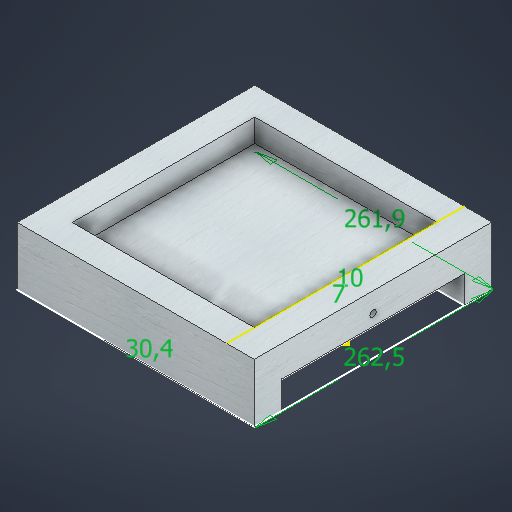
# Autodesk Inventor part: FundoColmeia
Saved by Autodesk Inventor 2027 (Build 310192000, 192)
## iProperties
Created: 2026-10-01
Part Number: FundoColmeia
Material: Genérico
Document SubType Name: Modeling
Designer: EspacoMaker
Density: 1 g/cm^3
Appearance: Padrão
Author: EspacoMaker
Autodesk Inventor part; units mm, degrees
ref_plane "YZ Plane" through (0, 0, 0) normal (1, 0, 0) x (0, 1, 0)
ref_plane "XZ Plane" through (0, 0, 0) normal (0, 1, 0) x (-1, 0, 0)
ref_plane "XY Plane" through (0, 0, 0) normal (0, 0, 1) x (1, 0, 0)
sketch "Esboço1" plane through (0, 0, 0) normal (0, 1, 0) x (-1, 0, 0)
  line L0 (130.95, 131.25) -> (-130.95, 131.25)
  line L1 (-130.95, 131.25) -> (-130.95, -131.25)
  line L2 (-130.95, -131.25) -> (130.95, -131.25)
  line L3 (130.95, -131.25) -> (130.95, 131.25)
  line L4 (130.95, 131.25) -> (-130.95, -131.25) construction
  line L5 (-130.95, 131.25) -> (130.95, -131.25) construction
  line L6 (-100.55, 100.85) -> (100.55, 100.85)
  line L7 (100.55, 100.85) -> (100.55, -100.85)
  line L8 (100.55, -100.85) -> (-100.55, -100.85)
  line L9 (-100.55, -100.85) -> (-100.55, 100.85)
  line L10 (100.55, 100.85) -> (130.95, 100.85)
  line L11 (-100.55, 100.85) -> (-130.95, 100.85)
  line L12 (100.55, -100.85) -> (130.95, -100.85)
  line L13 (-100.55, -100.85) -> (-130.95, -100.85)
  point P0 (0, 0)
  dimension "d0" = 261.9
  dimension "d1" = 262.5
  dimension "d2" = 30.4
  constraints: 28 end point, 6 point on line, 4 parallel, 4 perpendicular, 2 midpoint, 1 horizontal, 3 other
  measures "d0" distance of L2.end L1.end
  measures "d1" distance of L1.end L0.end
  measures "d2" distance between parallel lines of L0 L6
extrude "Extrusão1" add sketch "Esboço1" along normal blind 64.5
extrude "Extrusão2" cut sketch "Esboço1" along normal blind 30.4 contours L3 L12 L7 L10 | L11 L9 L13 L1 | L7 L8 L9 L6
sketch "Esboço2" plane through (0, 64.5, 0) normal (0, 1, 0) x (1, 0, 0)
  line L0 (130.95, 131.25) -> (-130.95, 131.25) projected
  line L1 (-130.95, 131.25) -> (-130.95, -131.25) projected
  line L2 (-130.95, -131.25) -> (130.95, -131.25) projected
  line L3 (130.95, -131.25) -> (130.95, 131.25) projected
  line L4 (130.95, -131.25) -> (130.95, 131.25) projected
  line L5 (100.55, 100.85) -> (100.55, -100.85) projected
  line L6 (100.55, -100.85) -> (-100.55, -100.85) projected
  line L7 (-100.55, -100.85) -> (-100.55, 100.85) projected
  line L8 (130.95, 100.85) -> (-130.95, 100.85) projected
  point P0 (0, 0)
extrude "Extrusão3" cut sketch "Esboço2" against normal blind 25.3 contours L5 L6 L7 L8
sketch "Esboço3" plane through (130.95, 0, -131.25) normal (1, 0, 0) x (0, 0, -1)
  line L0 (-232.1, 30.4) -> (-30.4, 30.4) projected
  line L1 (-131.25, 30.4) -> (-131.25, 64.5) construction
  line L2 (-262.5, 64.5) -> (0, 64.5) projected
  line L3 (-232.1, 0) -> (-232.1, 30.4) projected
  line L4 (-232.1, 30.4) -> (-30.4, 30.4) projected
  line L5 (-30.4, 30.4) -> (-30.4, 0) projected
  line L6 (-30.4, 0) -> (0, 0) projected
  line L7 (0, 0) -> (0, 64.5) projected
  line L8 (-262.5, 64.5) -> (0, 64.5) projected
  line L9 (-262.5, 0) -> (-262.5, 64.5) projected
  line L10 (-262.5, 0) -> (-232.1, 0) projected
  line L11 (-232.1, 39.2) -> (-30.4, 39.2) projected
  circle A0 centre (-131.25, 42.7) radius 3.5
  point P0 (-131.25, 0)
  dimension "d9" = 7
  constraints: 2 end point, 2 midpoint, 1 centre point, 1 point on line, 1 tangent
  measures "d9" diameter of A0
sketch "Esboço4" plane through (100.55, 64.5, -100.85) normal (-1, 0, 0) x (0, 0, 1)
  circle A0 centre (100.85, -21.8) radius 3.5 projected
  circle A1 centre (100.85, -10) radius 3.5
  line L0 (232.1, 0) -> (-30.4, 0) projected
  line L1 (100.85, 0) -> (100.85, -10) construction
  point P0 (100.85, -64.5)
  dimension "d10" = 7
  dimension "d11" = 10
  constraints: 2 end point, 1 centre point, 1 coincident, 1 midpoint, 1 vertical
  measures "d10" diameter of A1
  measures "d11" distance of L1.start L1.end
sketch3d "Esboço 3D1"
  line L0 (130.95, 42.7, 0) -> (100.55, 54.5, 0)
sweep "Varredura1" cut profiles "Esboço3" path "Esboço 3D1" contours A0
